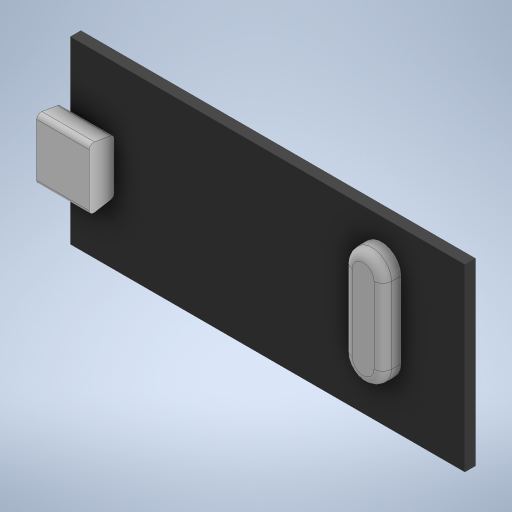
# Autodesk Inventor part: 블루투스 모듈
Saved by Autodesk Inventor 2023.1 (Build 271208000, 208)
## iProperties
Created: 2022-08-10
Part Number: 블루투스 모듈
Material: 일반
Document SubType Name: Modeling
Designer: fly01
Density: 1 g/cm^3
Appearance: 기본값
Author: fly01
Autodesk Inventor part; units mm, degrees
ref_plane "YZ Plane" through (0, 0, 0) normal (1, 0, 0) x (0, 1, 0)
ref_plane "XZ Plane" through (0, 0, 0) normal (0, 1, 0) x (-1, 0, 0)
ref_plane "XY Plane" through (0, 0, 0) normal (0, 0, 1) x (1, 0, 0)
sketch "스케치1" plane through (0, 0, 0) normal (0, 0, 1) x (1, 0, 0)
  line L0 (-22.5, -10.25) -> (22.5, -10.25)
  line L1 (22.5, -10.25) -> (22.5, 10.25)
  line L2 (22.5, 10.25) -> (-22.5, 10.25)
  line L3 (-22.5, 10.25) -> (-22.5, -10.25)
  line L4 (-22.5, -10.25) -> (22.5, 10.25) construction
  line L5 (22.5, -10.25) -> (-22.5, 10.25) construction
  point P0 (0, 0)
  dimension "d0" = 45
  dimension "d1" = 20.5
  constraints: 12 end point, 2 midpoint, 2 parallel, 1 horizontal, 1 perpendicular
  measures "d0" distance of L2.end L1.end
  measures "d1" distance of L1.end L0.end
extrude "돌출1" add sketch "스케치1" along normal blind 1.2
sketch "스케치2" plane through (-22.5, -10.25, 0) normal (-1, 0, 0) x (0, 0, 1)
  line L0 (1.2, 0) -> (1.2, 20.5) projected
  line L1 (4.05, 6.65) -> (1.2, 6.65) construction
  line L2 (1.2, 6.65) -> (1.2, 13.85)
  line L3 (1.2, 13.85) -> (4.05, 13.85) construction
  line L4 (4.05, 13.2546) -> (4.05, 7.2454)
  line L5 (4.05, 6.65) -> (1.2, 13.85) construction
  line L6 (1.2, 6.65) -> (4.05, 13.85) construction
  line L7 (1.6136, 13.4226) -> (3.4636, 13.7471)
  line L8 (1.6136, 7.0774) -> (3.4636, 6.7529)
  line L9 (1.2, 12.9301) -> (1.2, 7.5699)
  line L10 (3.85, 7.4835) -> (3.85, 13.0165)
  line L11 (3.2636, 13.509) -> (1.8136, 13.2546)
  line L12 (1.4, 12.7621) -> (1.4, 7.7379)
  line L13 (1.8136, 7.2454) -> (3.2636, 6.991)
  line L14 (2.375, 8.25) -> (2.875, 8.25)
  line L15 (2.875, 8.25) -> (2.875, 12.25)
  line L16 (2.875, 12.25) -> (2.375, 12.25)
  line L17 (2.375, 12.25) -> (2.375, 8.25)
  line L18 (2.375, 8.25) -> (2.875, 12.25) construction
  line L19 (2.875, 8.25) -> (2.375, 12.25) construction
  arc A0 (1.6136, 13.4226) -> (1.2, 12.9301) centre (1.7, 12.9301) ccw
  arc A1 (4.05, 13.2546) -> (3.4636, 13.7471) centre (3.55, 13.2546) ccw
  arc A2 (3.4636, 6.7529) -> (4.05, 7.2454) centre (3.55, 7.2454) ccw
  arc A3 (1.2, 7.5699) -> (1.6136, 7.0774) centre (1.7, 7.5699) ccw
  arc A4 (1.4, 7.7379) -> (1.8136, 7.2454) centre (1.9, 7.7379) ccw
  arc A5 (3.2636, 6.991) -> (3.85, 7.4835) centre (3.35, 7.4835) ccw
  arc A6 (3.85, 13.0165) -> (3.2636, 13.509) centre (3.35, 13.0165) ccw
  arc A7 (1.8136, 13.2546) -> (1.4, 12.7621) centre (1.9, 12.7621) ccw
  point P0 (0, 10.25)
  point P1 (2.625, 10.25)
  point P2 (1.2, 10.25)
  point P3 (1.2, 13.35)
  point P4 (1.2, 7.15)
  dimension "d4" = 2.85
  dimension "d5" = 7.2
  dimension "d6" = 0.5
  dimension "d7" = 0.5
  dimension "d8" = 0.2
  dimension "d9" = 0.5
  dimension "d10" = 4
  dimension "d11" = 0.5
  constraints: 38 end point, 16 point on circle, 16 tangent, 11 point on line, 8 centre point, 7 equal radius, 6 midpoint, 4 parallel, 2 horizontal, 2 perpendicular, 1 collinear, 3 other
  measures "d4" distance of L2.end L3.end
  measures "d5" distance of L3.end L1.start
  measures "d6" distance of L2.end point (1.2, 13.35)
  measures "d7" distance of L1.end point (1.2, 7.15)
  measures "d8" distance between parallel lines of L4 L10
  measures "d9" distance of L15.end L16.end
  measures "d10" distance of L14.end L15.end
  measures "d11" radius of A0
extrude "돌출2" add sketch "스케치2" along normal blind 1 and the other way blind 5
sketch "스케치3" plane through (-17.5, -10.25, 0) normal (1, 0, 0) x (0, 0, -1)
  arc A0 (-4.05, 7.2454) -> (-3.4636, 6.7529) centre (-3.55, 7.2454) ccw projected
  line L0 (-3.4636, 6.7529) -> (-1.6136, 7.0774) projected
  arc A1 (-1.6136, 7.0774) -> (-1.2, 7.5699) centre (-1.7, 7.5699) ccw projected
  line L1 (-1.2, 12.9301) -> (-1.2, 7.5699) projected
  arc A2 (-1.2, 12.9301) -> (-1.6136, 13.4226) centre (-1.7, 12.9301) ccw projected
  line L2 (-1.6136, 13.4226) -> (-3.4636, 13.7471) projected
  arc A3 (-3.4636, 13.7471) -> (-4.05, 13.2546) centre (-3.55, 13.2546) ccw projected
  line L3 (-4.05, 13.2546) -> (-4.05, 7.2454) projected
  arc A4 (-3.85, 7.4835) -> (-3.2636, 6.991) centre (-3.35, 7.4835) ccw projected
  line L4 (-3.85, 7.4835) -> (-3.85, 13.0165) projected
  arc A5 (-3.2636, 13.509) -> (-3.85, 13.0165) centre (-3.35, 13.0165) ccw projected
  line L5 (-3.2636, 13.509) -> (-1.8136, 13.2546) projected
  arc A6 (-1.4, 12.7621) -> (-1.8136, 13.2546) centre (-1.9, 12.7621) ccw projected
  line L6 (-1.4, 12.7621) -> (-1.4, 7.7379) projected
  arc A7 (-1.8136, 7.2454) -> (-1.4, 7.7379) centre (-1.9, 7.7379) ccw projected
  line L7 (-1.8136, 7.2454) -> (-3.2636, 6.991) projected
  point P0 (0, 10.25)
extrude "돌출3" add sketch "스케치3" against normal blind 1 contours L3 A3 L2 A2 L1 A1 L0 A0 | L4 A5 L5 A6 L6 A7 L7 A4
sketch "스케치4" plane through (0, 0, 1.2) normal (0, 0, 1) x (1, 0, 0)
  line L0 (12.9932, 5.5013) -> (12.9932, -3.185) construction
  line L1 (15.2371, 5.5013) -> (15.2371, -3.185)
  line L2 (10.7492, -3.185) -> (10.7492, 5.5013)
  arc A0 (15.2371, 5.5013) -> (10.7492, 5.5013) centre (12.9932, 5.5013) ccw
  arc A1 (10.7492, -3.185) -> (15.2371, -3.185) centre (12.9932, -3.185) ccw
  point P0 (0, 0)
  point P1 (12.9932, 1.1582)
  constraints: 8 end point, 4 point on circle, 4 tangent, 2 centre point, 1 midpoint, 1 parallel, 1 vertical
extrude "돌출4" add sketch "스케치4" along normal blind 2.1
fillet "모깎기1" radius 1 4 edges at (12.9932, 7.7452, 3.3) (10.7492, 1.1582, 3.3) (12.9932, -5.4289, 3.3) (15.2371, 1.1582, 3.3)
